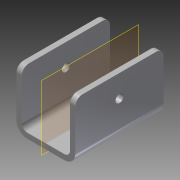
# Autodesk Inventor part: GE-13025-02
Saved by Autodesk Inventor 2013 (Build 170138000, 138)
## iProperties
Created: 2013-01-06
Part Number: GE-13025-02
Material: Steel
Document SubType Name: Modeling
Designer: Phillip
Density: 1 g/cm^3
Author: Phillip
Autodesk Inventor part; units mm, degrees
ref_plane "YZ Plane" through (0, 0, 0) normal (1, 0, 0) x (0, 1, 0)
ref_plane "XZ Plane" through (0, 0, 0) normal (0, 1, 0) x (-1, 0, 0)
ref_plane "XY Plane" through (0, 0, 0) normal (0, 0, 1) x (1, 0, 0)
sketch "Sketch1" plane through (0, 0, 0) normal (0, 0, 1) x (1, 0, 0)
  line L0 (9.398, 0) -> (41.402, 0)
  line L1 (50.8, 9.398) -> (50.8, 50.8)
  line L2 (50.8, 50.8) -> (46.228, 50.8)
  line L3 (46.228, 50.8) -> (46.228, 9.398)
  line L4 (41.402, 4.572) -> (9.398, 4.572)
  line L5 (4.572, 9.398) -> (4.572, 50.8)
  line L6 (4.572, 50.8) -> (0, 50.8)
  line L7 (0, 50.8) -> (0, 9.398)
  arc A0 (4.572, 9.398) -> (9.398, 4.572) centre (9.398, 9.398) ccw
  arc A1 (41.402, 4.572) -> (46.228, 9.398) centre (41.402, 9.398) ccw
  arc A2 (0, 9.398) -> (9.398, 0) centre (9.398, 9.398) ccw
  arc A3 (41.402, 0) -> (50.8, 9.398) centre (41.402, 9.398) ccw
  point P0 (0, 0)
  point P1 (50.8, 0)
  dimension "d0" = 50.8
  dimension "d1" = 50.8
  dimension "d2" = 4.572
  dimension "d3" = 4.572
  dimension "d4" = 4.572
  dimension "d5" = 4.826
  dimension "d6" = 9.398
  constraints: 16 end point, 8 point on circle, 8 tangent, 4 centre point, 4 perpendicular, 4 point on line, 3 parallel, 2 equal radius, 1 horizontal
  measures "d0" distance of point (0, 0) point (50.8, 0)
  measures "d1" distance of point (50.8, 0) L1.end
  measures "d2" distance of L1.end L2.end
  measures "d3" distance between parallel lines of L7 L5
  measures "d4" distance between parallel lines of L0 L4
  measures "d5" radius of A0
  measures "d6" radius of A2
extrude "Extrusion1" add sketch "Sketch1" against normal blind 76.2
fillet "Fillet1" radius 6.35 4 edges at (2.286, 50.8, 0) (48.514, 50.8, 0) (2.286, 50.8, -76.2) (48.514, 50.8, -76.2)
sketch "Sketch2" plane through (50.8, 9.398, 0) normal (1, 0, 0) x (0, 0, -1)
  line L0 (6.35, 41.402) -> (69.85, 41.402) projected
  line L1 (0, -9.398) -> (76.2, -9.398) projected
  point P0 (38.1, 22.352)
  point P1 (38.1, 41.402)
  dimension "d10" = 31.75
  constraints: 1 midpoint, 1 vertical alignment
  measures "d10" distance from line of point (38.1, 22.352) L1
hole "Hole1" at (50.8, 31.75, -38.1) direction (-1, 0, 0) diameter 6.858 end through all
ref_plane "Work Plane1" through (25.4, 9.398, 0) normal (1, 0, 0) x (0, 0, -1)
ref_plane "Work Plane2" through (0, 0, -38.1) normal (0, 0, -1) x (-1, 0, 0)
equation "\"d3\" = d2"
equation "\"d4\" = d2"
body "Solid1"
